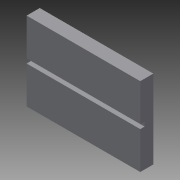
# Autodesk Inventor part: 000106
Saved by Autodesk Inventor 2015 (Build 190159000, 159)
## iProperties
Created: 2015-05-12
Part Number: 000106
Material: Generic
Document SubType Name: Modeling
Designer: Wesley
Density: 1 g/cm^3
Appearance: Default
Author: Wesley
Autodesk Inventor part; units mm, degrees
ref_plane "YZ Plane" through (0, 0, 0) normal (1, 0, 0) x (0, 1, 0)
ref_plane "XZ Plane" through (0, 0, 0) normal (0, 1, 0) x (-1, 0, 0)
ref_plane "XY Plane" through (0, 0, 0) normal (0, 0, 1) x (1, 0, 0)
sketch "Sketch1" plane through (0, 0, 0) normal (0, 0, 1) x (1, 0, 0)
  line L0 (0, 0) -> (82.55, 0)
  line L1 (82.55, 0) -> (82.55, 57.15)
  line L2 (82.55, 57.15) -> (0, 57.15)
  line L3 (0, 57.15) -> (0, 0)
  dimension "d0" = 57.15
  dimension "d1" = 82.55
  constraints: 8 end point, 2 parallel, 1 horizontal, 1 perpendicular
  measures "d0" distance of L2.end L0.start
  measures "d1" distance of L0.start L0.end
extrude "Extrusion1" add sketch "Sketch1" along normal blind 9.525
sketch "Sketch2" plane through (0, 0, 9.525) normal (0, 0, 1) x (1, 0, 0)
  line L0 (-21.536, 28.575) -> (122.8285, 28.575) construction
  line L1 (82.55, 57.15) -> (0, 57.15) construction
  line L2 (0, 57.15) -> (0, 0) projected
  line L3 (82.55, 0) -> (82.55, 57.15) projected
  line L4 (0, 26.9875) -> (82.55, 26.9875)
  line L5 (82.55, 26.9875) -> (82.55, 30.1625)
  line L6 (82.55, 30.1625) -> (0, 30.1625)
  line L7 (0, 30.1625) -> (0, 26.9875)
  dimension "d4" = 28.575
  dimension "d5" = 1.5875
  dimension "d6" = 1.5875
  constraints: 10 end point, 2 horizontal, 2 parallel, 2 point on line, 1 perpendicular
  measures "d4" distance between parallel lines of L1 L0
  measures "d5" distance between parallel lines of L4 L0
  measures "d6" distance between parallel lines of L6 L0
extrude "Extrusion2" cut sketch "Sketch2" against normal blind 3.175
body "Solid1"
